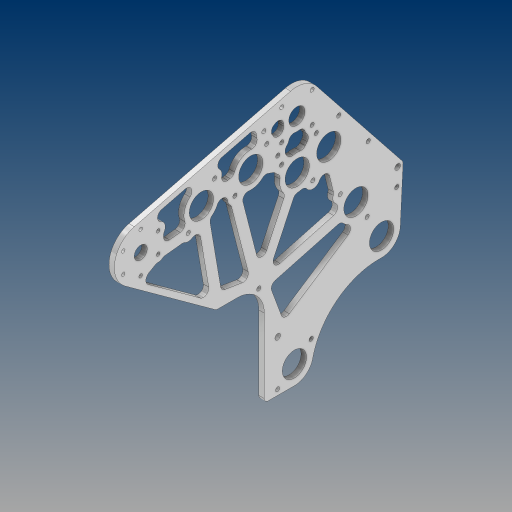
# Autodesk Inventor part: Intake Roller Plate
Saved by Autodesk Inventor 2024.3 (Build 283343000, 343)
## iProperties
Created: 2024-07-25
Part Number: Intake Roller Plate
Material: Aluminum 6061
Document SubType Name: Modeling
Designer: Kenji
Density: 2.7 g/cm^3
Appearance: Aluminum - Dark
Mass: 571.226 g
Surface Area: 904.797 cm^2
Volume: 211.565 cm^3
Author: Kenji
Autodesk Inventor part; units mm, degrees
ref_plane "YZ Plane" through (0, 0, 0) normal (1, 0, 0) x (0, 1, 0)
ref_plane "XZ Plane" through (0, 0, 0) normal (0, 1, 0) x (-1, 0, 0)
ref_plane "XY Plane" through (0, 0, 0) normal (0, 0, 1) x (1, 0, 0)
sketch "Sketch1" plane through (0, 0, 0) normal (1, 0, 0) x (0, 1, 0)
  line L0 (127, 0) -> (127, -31.75) construction
  line L1 (95.25, -63.5) -> (31.75, -63.5) construction
  line L2 (0, -31.75) -> (0, 0) construction
  arc A0 (95.25, -63.5) -> (127, -31.75) centre (95.25, -31.75) ccw construction
  arc A1 (0, -31.75) -> (31.75, -63.5) centre (31.75, -31.75) ccw construction
  line L3 (0, 0) -> (0, 19.05) construction
  line L4 (0, 19.05) -> (-12.7, 19.05) construction
  line L5 (82.55, 19.05) -> (82.55, 292.1) construction
  circle A2 centre (82.55, 292.1) radius 25.4 construction
  circle A3 centre (82.55, 292.1) radius 31.75 construction
  circle A4 centre (231.775, 292.1) radius 25.4 construction
  circle A5 centre (231.775, 292.1) radius 31.75 construction
  line L6 (-12.7, 19.05) -> (82.55, 19.05) construction
  line L7 (127, 0) -> (0, 0) construction
  line L8 (-12.7, 19.05) -> (-12.7, -285.75) construction
  circle A6 centre (38.1, -172.5837) radius 50.8 construction
  circle A7 centre (104.9083, -202.0677) radius 25.4 construction
  circle A8 centre (104.9083, -202.0677) radius 14.2875
  circle A9 centre (154.8209, -171.8196) radius 25.4 construction
  circle A10 centre (154.8209, -171.8196) radius 14.2875
  circle A11 centre (250.0002, -47.5843) radius 22.225 construction
  circle A12 centre (250.0002, -47.5843) radius 25.4 construction
  circle A13 centre (250.0002, -47.5843) radius 14.2875
  line L9 (82.55, 19.05) -> (127, 19.05) construction
  line L10 (127, 19.05) -> (127, 0) construction
  circle A14 centre (154.8209, -171.8196) radius 22.225 construction
  circle A15 centre (104.9083, -202.0677) radius 22.225 construction
  circle A16 centre (25.4, -99.06) radius 25.4 construction
  circle A17 centre (25.4, -99.06) radius 23.8125 construction
  line L11 (25.4, -73.66) -> (25.4, -63.5) construction
  circle A18 centre (219.8086, -102.3786) radius 25.4 construction
  circle A19 centre (219.8086, -102.3786) radius 22.225 construction
  circle A20 centre (219.8086, -102.3786) radius 14.2875
  line L12 (0, -99.06) -> (-12.7, -99.06) construction
  circle A21 centre (63.172, -79.375) radius 6.477 construction
  circle A22 centre (25.4, -99.06) radius 14.2875
  circle A23 centre (63.172, -79.375) radius 3.2512
  circle A24 centre (95.1707, -129.6948) radius 50.8 construction
  circle A25 centre (147.0613, -96.0158) radius 50.8 construction
  circle A26 centre (105.4747, -117.9903) radius 50.8 construction
  circle A27 centre (166.1747, -221.0415) radius 3.2512
  circle A28 centre (242.3971, 10.8357) radius 14.2875
  circle A29 centre (242.3971, 10.8357) radius 22.225 construction
  line L13 (219.8086, -102.3786) -> (154.8209, -171.8196) construction
  line L14 (154.8209, -171.8196) -> (104.9083, -202.0677) construction
  line L15 (82.55, 19.05) -> (31.75, 19.05) construction
  line L16 (31.75, 19.05) -> (31.75, 292.1) construction
  line L17 (31.75, 292.1) -> (82.55, 292.1) construction
  circle A30 centre (242.3971, 10.8357) radius 7.62 construction
  line L18 (-12.7, -285.75) -> (571.5, -285.75) construction
  line L19 (571.5, -285.75) -> (571.5, 292.1) construction
  line L20 (31.75, 292.1) -> (571.5, 292.1) construction
  line L21 (127, 19.05) -> (571.5, 19.05) construction
  circle A31 centre (230.3321, 82.55) radius 7.62
  circle A32 centre (230.3321, 82.55) radius 23.8125 construction
  circle A33 centre (254.1446, 82.55) radius 2.0828
  circle A34 centre (230.3321, 82.55) radius 27.94 construction
  circle A35 centre (230.3321, 82.55) radius 31.115 construction
  circle A36 centre (242.2384, 103.1722) radius 2.0828
  circle A37 centre (218.4259, 103.1722) radius 2.0828
  circle A38 centre (206.5196, 82.55) radius 2.0828
  circle A39 centre (218.4259, 61.9278) radius 2.0828
  circle A40 centre (242.2384, 61.9278) radius 2.0828
  line L22 (-12.7, -63.5) -> (368.3, -63.5) construction
  circle A41 centre (166.1747, -221.0415) radius 6.4262 construction
  line L23 (368.3, -63.5) -> (368.3, -285.75) construction
  circle A42 centre (63.172, -79.375) radius 6.35 construction
  circle A43 centre (242.3971, 10.8357) radius 25.4 construction
  line L24 (242.3971, 10.8357) -> (250.0002, -47.5843) construction
  line L25 (82.55, 19.05) -> (141.3002, 19.05) construction
  line L26 (141.3002, 19.05) -> (141.3002, 209.55) construction
  line L27 (141.3002, 209.55) -> (82.55, 209.55) construction
  line L28 (82.55, 209.55) -> (82.55, 19.05) construction
  circle A44 centre (133.35, 12.7) radius 6.35 construction
  circle A45 centre (177.4795, -39.017) radius 50.8 construction
  circle A46 centre (177.8, -23.221) radius 50.8 construction
  circle A47 centre (25.4, -99.06) radius 22.225 construction
  line L29 (3.175, -99.06) -> (3.175, -68.2752)
  circle A48 centre (133.35, 12.7) radius 3.2512 construction
  arc A49 (166.1747, -227.4677) -> (170.1786, -226.0679) centre (166.1747, -221.0415) ccw
  arc A50 (3.175, -99.06) -> (20.3984, -120.7149) centre (25.4, -99.06) ccw
  arc A51 (7.9502, -63.5) -> (3.175, -68.2752) centre (7.9502, -68.2752) ccw
  arc A52 (260.5134, 90.1152) -> (205.1617, 100.8419) centre (230.3321, 82.55) ccw
  line L30 (141.3002, 53.086) -> (157.9626, 53.086) construction
  line L31 (157.9626, 53.086) -> (157.9626, 86.106) construction
  line L32 (157.9626, 86.106) -> (141.3002, 86.106) construction
  line L33 (141.3002, 86.106) -> (141.3002, 53.086) construction
  line L34 (232.868, -28.832) -> (267.1324, -66.3365) construction
  circle A53 centre (232.868, -28.832) radius 2.4257
  circle A54 centre (267.1324, -66.3365) radius 2.4257
  line L35 (236.3587, 15.4834) -> (262.5254, -4.6567) construction
  line L36 (236.3587, 15.4834) -> (222.2689, 26.3281) construction
  circle A55 centre (262.5254, -4.6567) radius 2.4257
  circle A56 centre (222.2689, 26.3281) radius 2.4257
  circle A57 centre (262.5254, -4.6567) radius 6.35 construction
  circle A58 centre (222.2689, 26.3281) radius 6.35 construction
  circle A59 centre (232.868, -28.832) radius 6.35 construction
  circle A60 centre (267.1324, -66.3365) radius 6.35 construction
  line L37 (219.8086, -102.3786) -> (237.1646, -83.8332) construction
  line L38 (219.8086, -102.3786) -> (202.4526, -120.9239) construction
  circle A61 centre (237.1646, -83.8332) radius 2.4257
  circle A62 centre (202.4526, -120.9239) radius 2.4257
  circle A63 centre (172.1769, -153.2743) radius 2.4257
  circle A64 centre (133.0985, -184.9838) radius 2.4257
  arc A65 (82.6927, -201.4208) -> (103.7686, -224.2634) centre (104.9083, -202.0677) ccw
  circle A66 centre (9.525, -79.2321) radius 2.4257
  circle A67 centre (9.525, -79.2321) radius 6.35 construction
  arc A68 (82.6927, -201.4208) -> (20.3984, -120.7149) centre (2.2987, -199.0799) ccw
  line L39 (9.525, -79.2321) -> (41.275, -118.8879) construction
  circle A69 centre (41.275, -118.8879) radius 2.4257
  circle A70 centre (41.275, -118.8879) radius 5.6007 construction
  line L40 (7.9502, -63.5) -> (95.25, -63.5)
  arc A71 (95.25, -63.5) -> (127, -31.75) centre (95.25, -31.75) ccw
  line L41 (166.1747, -227.4677) -> (103.7686, -224.2634)
  line L42 (104.9083, -202.0677) -> (83.1859, -215.2319) construction
  line L43 (82.55, 133.35) -> (88.9, 133.35) construction
  line L44 (82.55, 184.15) -> (88.9, 184.15) construction
  line L45 (127, -31.75) -> (127, -8.2637)
  line L46 (127.9123, -5.4564) -> (205.1617, 100.8419)
  arc A72 (127.9123, -5.4564) -> (127, -8.2637) centre (131.7752, -8.2637) ccw
  line L47 (82.55, 44.45) -> (571.5, 44.45) construction
  circle A73 centre (133.0985, -184.9838) radius 6.35 construction
  circle A74 centre (141.7169, -99.98) radius 50.8 construction
  circle A75 centre (277.7476, -102.0288) radius 30 construction
  circle A76 centre (277.7476, -102.0288) radius 25.4 construction
  circle A77 centre (303.1476, -102.0288) radius 2.3876 construction
  circle A78 centre (295.7081, -84.0683) radius 2.3876
  circle A79 centre (277.7476, -76.6288) radius 2.3876 construction
  circle A80 centre (259.7871, -84.0683) radius 2.3876
  circle A81 centre (252.3476, -102.0288) radius 2.3876 construction
  circle A82 centre (259.7871, -119.9893) radius 2.3876
  circle A83 centre (277.7476, -127.4288) radius 2.3876 construction
  circle A84 centre (295.7081, -119.9893) radius 2.3876
  circle A85 centre (277.7476, -102.0288) radius 9.525
  circle A86 centre (219.8086, -102.3786) radius 19.05 construction
  circle A87 centre (227.4601, -139.7023) radius 19.05 construction
  circle A88 centre (227.4601, -139.7023) radius 14.2875
  line L48 (247.7482, -102.2099) -> (245.2082, -102.2252) construction
  line L49 (170.1786, -226.0679) -> (296.4391, -125.4942)
  line L50 (260.5134, 90.1152) -> (306.8474, -94.7347)
  arc A89 (296.4391, -125.4942) -> (306.8474, -94.7347) centre (277.7476, -102.0288) ccw
  circle A90 centre (219.8086, -102.3786) radius 30.48 construction
  circle A91 centre (277.7476, -102.0288) radius 30.48 construction
  circle A92 centre (248.6408, -79.4624) radius 3.81 construction
  line L51 (251.6519, -81.7968) -> (253.6592, -83.3531) construction
  line L52 (245.6582, -81.833) -> (243.6698, -83.4134) construction
  circle A93 centre (248.6408, -79.4624) radius 2.3812
  circle A94 centre (248.9154, -124.945) radius 3.81 construction
  circle A95 centre (248.9154, -124.945) radius 2.3876
  line L53 (251.898, -122.5744) -> (253.8865, -120.9939) construction
  line L54 (245.9043, -122.6105) -> (243.897, -121.0542) construction
  line L55 (248.6408, -75.6524) -> (248.6408, -72.9479) construction
  line L56 (219.8086, -102.3786) -> (219.8086, -88.0911) construction
  circle A96 centre (232.868, -28.832) radius 2.4257
  circle A97 centre (9.525, -79.2321) radius 2.4257
  circle A98 centre (146.08, -220.0775) radius 2.4257
  circle A99 centre (253.6387, -151.4689) radius 2.4257
  circle A100 centre (209.9304, -186.285) radius 2.4257
  circle A101 centre (281.6771, -62.9926) radius 2.4257
  line L57 (123.7263, -57.0623) -> (232.868, -28.832) construction
  line L58 (232.868, -28.832) -> (281.6771, -62.9926) construction
  line L59 (281.6771, -62.9926) -> (253.6387, -151.4689) construction
  line L60 (253.6387, -151.4689) -> (209.9304, -186.285) construction
  line L61 (209.9304, -186.285) -> (146.08, -220.0775) construction
  line L62 (146.08, -220.0775) -> (9.525, -79.2321) construction
  line L63 (123.7263, -57.0623) -> (9.525, -79.2321) construction
  circle A102 centre (146.08, -220.0775) radius 6.35 construction
  circle A103 centre (123.7263, -57.0623) radius 2.4257
  line L64 (277.7476, -102.0288) -> (219.8086, -102.3786) construction
  line L65 (250.0002, -47.5843) -> (219.8086, -102.3786) construction
  point P0 (-12.7, -172.5837)
  point P1 (180.2209, -171.8196)
  point P2 (104.775, 19.05)
  point P3 (172.6009, -221.0415)
  point P4 (127, -63.5)
  point P5 (3.175, -63.5)
  point P6 (104.9083, -227.4677)
  point P7 (95.25, -63.5)
  point P8 (127, -6.7118)
  point P9 (222.7121, 82.55)
  point P10 (220.1721, 10.8357)
  point P11 (25.4, -99.06)
  dimension "d58" = 101.6
  dimension "d267" = 15.24
  dimension "d283" = 15.24
  dimension "d284" = 47.625
  dimension "d523" = 50.8
  dimension "d2" = 31.75
  dimension "d3" = 19.05
  dimension "d4" = 12.7
  dimension "d7" = 273.05
  dimension "d8" = 50.8
  dimension "d9" = 6.35
  dimension "d10" = 50.8
  dimension "d11" = 6.35
  dimension "d12" = 149.225
  dimension "d14" = 127
  dimension "d16" = 304.8
  dimension "d175" = 31.75
  dimension "d180" = 50.8
  dimension "d181" = 1.5875
  dimension "d187" = 31.75
  dimension "d189" = 12.7
  dimension "d191" = 12.954
  dimension "d192" = 28.575
  dimension "d201" = 6.5024
  dimension "d207" = 101.6
  dimension "d208" = 101.6
  dimension "d210" = 130.175
  dimension "d214" = 15.875
  dimension "d218" = 6.5024
  dimension "d220" = 143.1895
  dimension "d236" = 50.8
  dimension "d237" = 44.45
  dimension "d271" = 584.2
  dimension "d285" = 4.1656
  dimension "d290" = 55.88
  dimension "d292" = 3.175
  dimension "d321" = 360
  dimension "d323" = 381
  dimension "d328" = 3.175
  dimension "d336" = 12.7
  dimension "d375" = 10.16
  dimension "d388" = 50.8
  dimension "d389" = 3.175
  dimension "d395" = 44.45
  dimension "d399" = 58.7502
  dimension "d400" = 190.5
  dimension "d404" = 12.7
  dimension "d405" = 101.6
  dimension "d406" = 101.6
  dimension "d409" = 3.175
  dimension "d410" = 6.5024
  dimension "d411" = 4.7752
  dimension "d427" = 16.6624
  dimension "d428" = 33.02
  dimension "d429" = 34.036
  dimension "d433" = 4.8514
  dimension "d434" = 4.8514
  dimension "d435" = 4.8514
  dimension "d436" = 4.8514
  dimension "d441" = 45
  dimension "d443" = 4.8514
  dimension "d444" = 4.8514
  dimension "d445" = 4.8514
  dimension "d446" = 4.8514
  dimension "d453" = 4.8514
  dimension "d459" = 4.8514
  dimension "d460" = 3.175
  dimension "d470" = 273.05
  dimension "d471" = 62.5615
  constraints: 133 end point, 97 centre point, 60 point on circle, 38 tangent, 36 point on line, 29 coincident, 16 equal radius, 16 perpendicular, 14 horizontal alignment, 12 concentric, 6 collinear, 6 horizontal, 6 parallel, 6 vertical, 5 midpoint, 4 equal length, 3 vertical alignment, 53 other
  measures "d2" radius of A0
  measures "d3" distance of L2.end L3.end
  measures "d4" distance of L3.end L4.end
  measures "d7" distance of L5.start L5.end
  measures "d8" diameter of A2
  measures "d9" radial gap between concentric circles of A2 A3
  measures "d10" diameter of A4
  measures "d11" radial gap between concentric circles of A4 A5
  measures "d12" distance of L17.end A4.centre
  measures "d14" distance of L0.start L2.end
  measures "d16" distance of L4.end L8.end
  measures "d175" radius of A1
  measures "d180" diameter of A16
  measures "d181" radial gap between concentric circles of A16 A17
  measures "d187" distance of L0.start L0.end
  measures "d189" distance of L12.start L12.end
  measures "d191" diameter of A21
  measures "d192" diameter of A22
  measures "d201" diameter of A23
  measures "d207" diameter of A24
  measures "d208" diameter of A25
  measures "d210" distance of A21.centre A14.centre
  measures "d214" distance from line of L1 A21.centre
  measures "d218" diameter of A27
  measures "d220" distance of A0.centre A19.centre
  measures "d236" distance of L5.start L15.end
  measures "d237" distance of L4.end L15.end
  measures "d271" distance of L8.end L18.end
  measures "d285" diameter of A33
  measures "d290" diameter of A34
  measures "d292" radial gap between concentric circles of A34 A35
  measures "d323" distance of L22.start L22.end
  measures "d328" radial gap between concentric circles of A27 A41
  measures "d336" diameter of A42
  measures "d375" distance of L11.start L11.end
  measures "d388" diameter of A9
  measures "d389" radial gap between concentric circles of A15 A7
  measures "d395" diameter of A15
  measures "d399" distance of L27.end L26.end
  measures "d400" distance of L26.end L25.end
  measures "d404" diameter of A44
  measures "d405" diameter of A45
  measures "d406" diameter of A46
  measures "d409" radial gap between concentric circles of A16 A47
  measures "d410" diameter of A48
  measures "d411" radius of A51
  measures "d427" distance of L32.end L31.end
  measures "d428" distance between parallel lines of L30 L32
  measures "d429" distance from line of L25.end L30
  measures "d433" diameter of A53
  measures "d434" diameter of A54
  measures "d435" diameter of A55
  measures "d436" diameter of A56
  measures "d441" angle of L24 L35
  measures "d443" diameter of A61
  measures "d444" diameter of A62
  measures "d445" diameter of A63
  measures "d446" diameter of A64
  measures "d453" diameter of A66
  measures "d459" diameter of A69
  measures "d460" radial gap between concentric circles of A69 A70
  measures "d470" distance of L19.end L21.end
  measures "d471" distance of A19.centre A11.centre
extrude "Extrusion14" add sketch "Sketch1" along normal blind 6.35 contours L29 A51 L40 A71 L45 A72 L46 A52 L50 A89 L49 A49 L41 A65 A68 A50 | A93 | A95 | A98 | A99 | A100 | A101 | A103
extrude "Extrusion16" cut sketch "Sketch1" along normal blind 6.35 contours A93 | A95
extrude "Extrusion17" cut sketch "Sketch1" along normal blind 25.4 contours A98 | A99 | A100 | A101 | A103
sketch "Sketch3" plane through (6.35, 0, 0) normal (1, 0, 0) x (0, 0, -1)
  circle A0 centre (151.4689, 253.6387) radius 2.4257 construction
  circle A1 centre (186.285, 209.9304) radius 2.4257 construction
  circle A2 centre (62.9926, 281.6771) radius 2.4257 construction
  circle A3 centre (220.0775, 146.08) radius 2.4257 construction
  circle A4 centre (57.0623, 123.7263) radius 2.4257 construction
  circle A5 centre (124.945, 248.9154) radius 2.3876 construction
  circle A6 centre (79.4624, 248.6408) radius 2.3812 construction
  line L0 (224.2634, 103.7686) -> (227.4677, 166.1747) projected
  arc A7 (227.4677, 166.1747) -> (226.0679, 170.1786) centre (221.0415, 166.1747) ccw projected
  line L1 (226.0679, 170.1786) -> (125.4942, 296.4391) projected
  arc A8 (125.4942, 296.4391) -> (94.7347, 306.8474) centre (102.0288, 277.7476) ccw projected
  line L2 (94.7347, 306.8474) -> (-90.1152, 260.5134) projected
  arc A9 (-90.1152, 260.5134) -> (-100.8419, 205.1617) centre (-82.55, 230.3321) ccw projected
  line L3 (-100.8419, 205.1617) -> (5.4564, 127.9123) projected
  arc A10 (5.4564, 127.9123) -> (8.2637, 127) centre (8.2637, 131.7752) ccw projected
  line L4 (8.2637, 127) -> (31.75, 127) projected
  arc A11 (63.5, 95.25) -> (31.75, 127) centre (31.75, 95.25) ccw projected
  line L5 (63.5, 95.25) -> (63.5, 7.9502) projected
  arc A12 (63.5, 7.9502) -> (68.2752, 3.175) centre (68.2752, 7.9502) ccw projected
  line L6 (68.2752, 3.175) -> (99.06, 3.175) projected
  arc A13 (99.06, 3.175) -> (120.7149, 20.3984) centre (99.06, 25.4) ccw projected
  arc A14 (201.4208, 82.6927) -> (120.7149, 20.3984) centre (199.0799, 2.2987) ccw projected
  arc A15 (201.4208, 82.6927) -> (224.2634, 103.7686) centre (202.0677, 104.9083) ccw projected
  circle A16 centre (119.9893, 259.7871) radius 2.3876 construction
  circle A17 centre (79.2321, 9.525) radius 2.4257 construction
  circle A18 centre (120.9239, 202.4526) radius 2.4257 construction
  circle A19 centre (-26.3281, 222.2689) radius 2.4257 construction
  circle A20 centre (28.832, 232.868) radius 2.4257 construction
  circle A21 centre (-61.9278, 242.2384) radius 2.0828 construction
  circle A22 centre (-61.9278, 218.4259) radius 2.0828 construction
  circle A23 centre (-82.55, 254.1446) radius 2.0828 construction
  circle A24 centre (-10.8357, 242.3971) radius 14.2875 construction
  circle A25 centre (79.375, 63.172) radius 3.2512 construction
  circle A26 centre (102.3786, 219.8086) radius 14.2875 construction
  circle A27 centre (171.8196, 154.8209) radius 14.2875 construction
  circle A28 centre (66.3365, 267.1324) radius 2.4257 construction
  circle A29 centre (83.8332, 237.1646) radius 2.4257 construction
  circle A30 centre (184.9838, 133.0985) radius 2.4257 construction
  circle A31 centre (118.8879, 41.275) radius 2.4257 construction
  circle A32 centre (139.7023, 227.4601) radius 14.2875 construction
  circle A33 centre (102.0288, 277.7476) radius 9.525 construction
  circle A34 centre (119.9893, 295.7081) radius 2.3876 construction
  circle A35 centre (84.0683, 259.7871) radius 2.3876 construction
  circle A36 centre (84.0683, 295.7081) radius 2.3876 construction
  circle A37 centre (153.2743, 172.1769) radius 2.4257 construction
  circle A38 centre (4.6567, 262.5254) radius 2.4257 construction
  circle A39 centre (-82.55, 206.5196) radius 2.0828 construction
  circle A40 centre (-103.1722, 218.4259) radius 2.0828 construction
  circle A41 centre (-103.1722, 242.2384) radius 2.0828 construction
  circle A42 centre (-82.55, 230.3321) radius 7.62 construction
  circle A43 centre (221.0415, 166.1747) radius 3.2512 construction
  circle A44 centre (99.06, 25.4) radius 14.2875 construction
  circle A45 centre (47.5843, 250.0002) radius 14.2875 construction
  circle A46 centre (202.0677, 104.9083) radius 14.2875 construction
  line L7 (120.5274, 292.4828) -> (221.1011, 166.2222) construction
  arc A47 (221.1109, 166.2061) -> (221.1011, 166.2222) centre (221.0415, 166.1747) ccw construction
  line L8 (221.1109, 166.2061) -> (217.9218, 104.0943) construction
  arc A48 (201.6056, 89.04) -> (217.9218, 104.0943) centre (202.0677, 104.9083) ccw construction
  arc A49 (201.6056, 89.04) -> (114.5278, 21.8275) centre (199.0799, 2.2987) ccw construction
  arc A50 (99.06, 9.525) -> (114.5278, 21.8275) centre (99.06, 25.4) ccw construction
  line L9 (99.06, 9.525) -> (69.85, 9.525) construction
  line L10 (69.85, 9.525) -> (69.85, 95.25) construction
  arc A51 (69.85, 95.25) -> (31.75, 133.35) centre (31.75, 95.25) ccw construction
  line L11 (31.75, 133.35) -> (8.7754, 133.35) construction
  line L12 (8.7754, 133.35) -> (-97.1089, 210.2985) construction
  arc A52 (-88.5712, 254.354) -> (-97.1089, 210.2985) centre (-82.55, 230.3321) ccw construction
  line L13 (-88.5712, 254.354) -> (96.2786, 300.6879) construction
  arc A53 (120.5274, 292.4828) -> (96.2786, 300.6879) centre (102.0288, 277.7476) ccw construction
  circle A54 centre (4.6567, 262.5254) radius 8.7757 construction
  circle A55 centre (-10.8357, 242.3971) radius 20.6375 construction
  circle A56 centre (-26.3281, 222.2689) radius 8.7757 construction
  circle A57 centre (-61.9278, 242.2384) radius 8.4328 construction
  circle A58 centre (-82.55, 254.1446) radius 8.4328 construction
  circle A59 centre (-61.9278, 218.4259) radius 8.4328 construction
  circle A60 centre (-82.55, 230.3321) radius 13.97 construction
  circle A61 centre (-82.55, 206.5196) radius 8.4328 construction
  circle A62 centre (-103.1722, 218.4259) radius 8.4328 construction
  circle A63 centre (-103.1722, 242.2384) radius 8.4328 construction
  circle A64 centre (47.5843, 250.0002) radius 20.6375 construction
  circle A65 centre (28.832, 232.868) radius 8.7757 construction
  circle A66 centre (62.9926, 281.6771) radius 8.7757 construction
  circle A67 centre (66.3365, 267.1324) radius 8.7757 construction
  circle A68 centre (102.0288, 277.7476) radius 15.875 construction
  circle A69 centre (84.0683, 259.7871) radius 8.7376 construction
  circle A70 centre (79.4624, 248.6408) radius 8.7312 construction
  circle A71 centre (83.8332, 237.1646) radius 8.7757 construction
  circle A72 centre (102.3786, 219.8086) radius 20.6375 construction
  circle A73 centre (120.9239, 202.4526) radius 8.7757 construction
  circle A74 centre (139.7023, 227.4601) radius 20.6375 construction
  circle A75 centre (124.945, 248.9154) radius 8.7376 construction
  circle A76 centre (119.9893, 259.7871) radius 8.7376 construction
  circle A77 centre (84.0683, 295.7081) radius 8.7376 construction
  circle A78 centre (119.9893, 295.7081) radius 8.7376 construction
  circle A79 centre (153.2743, 172.1769) radius 8.7757 construction
  circle A80 centre (171.8196, 154.8209) radius 20.6375 construction
  circle A81 centre (184.9838, 133.0985) radius 8.7757 construction
  circle A82 centre (57.0623, 123.7263) radius 8.7757 construction
  circle A83 centre (79.375, 63.172) radius 9.6012 construction
  line L14 (90.2467, 265.9655) -> (90.8035, 266.5223) construction
  line L15 (113.8109, 265.9655) -> (113.2541, 266.5223) construction
  line L16 (119.5913, 242.0101) -> (115.0235, 236.1184) construction
  line L17 (114.178, 245.3915) -> (111.9505, 242.5184)
  arc A84 (99.5909, 262.0609) -> (104.4667, 262.0609) centre (102.0288, 277.7476) ccw
  arc A85 (105.8607, 240.1502) -> (97.5577, 239.8752) centre (102.3786, 219.8086) ccw
  arc A86 (116.6652, 251.7065) -> (116.2491, 248.0628) centre (124.945, 248.9154) ccw construction
  arc A87 (111.5645, 257.4701) -> (113.7175, 253.7035) centre (119.9893, 259.7871) ccw
  arc A88 (90.1332, 253.4973) -> (92.4931, 257.4701) centre (84.0683, 259.7871) ccw
  arc A89 (88.182, 248.1918) -> (88.192, 248.806) centre (79.4624, 248.6408) ccw
  arc A90 (90.9354, 242.3195) -> (90.0356, 243.3729) centre (83.8332, 237.1646) ccw
  arc A91 (90.1332, 253.4973) -> (88.192, 248.806) centre (94.5409, 248.9262) ccw
  arc A92 (88.182, 248.1918) -> (90.0356, 243.3729) centre (94.5236, 247.8652) ccw
  arc A93 (90.9354, 242.3195) -> (97.5577, 239.8752) centre (96.0744, 246.0495) ccw
  arc A94 (105.8607, 240.1502) -> (111.9505, 242.5184) centre (106.9321, 246.4092) ccw
  arc A95 (114.178, 245.3915) -> (113.7175, 253.7035) centre (109.1596, 249.2822) ccw
  circle A96 centre (105.4418, 255.7862) radius 6.35 construction
  arc A97 (111.5645, 257.4701) -> (104.4667, 262.0609) centre (105.4418, 255.7862) ccw
  circle A98 centre (98.6158, 255.7862) radius 6.35 construction
  arc A99 (99.5909, 262.0609) -> (92.4931, 257.4701) centre (98.6158, 255.7862) ccw
  line L18 (144.6227, 207.4178) -> (151.182, 180.6995) construction
  line L19 (93.5751, 201.143) -> (60.8058, 131.6635) construction
  line L20 (87.3804, 68.4726) -> (177.6667, 128.2536) construction
  line L21 (76.0554, 72.1811) -> (60.0965, 115.4918) construction
  line L22 (97.964, 195.5626) -> (74.5331, 145.8831)
  line L23 (140.6011, 197.1653) -> (145.1487, 178.6417)
  line L24 (126.1934, 209.4701) -> (127.3102, 210.9574) construction
  arc A100 (103.3946, 199.1961) -> (107.1994, 199.7421) centre (102.3786, 219.8086) ccw
  arc A101 (113.8218, 197.2978) -> (128.7624, 198.5066) centre (120.9239, 202.4526) ccw
  arc A102 (113.8218, 197.2978) -> (107.1994, 199.7421) centre (108.6827, 193.5678) ccw
  arc A103 (103.3946, 199.1961) -> (97.964, 195.5626) centre (103.7073, 192.8538) ccw
  circle A104 centre (134.4342, 195.6513) radius 6.35 construction
  arc A105 (140.6011, 197.1653) -> (128.7624, 198.5066) centre (134.4342, 195.6513) ccw
  line L25 (151.9004, 149.4236) -> (65.5325, 126.0214) construction
  line L26 (150.4966, 142.4643) -> (76.4793, 122.4086)
  line L27 (93.1071, 79.8802) -> (162.4617, 125.8018)
  line L28 (83.643, 82.9793) -> (72.1817, 114.0841)
  arc A106 (76.4793, 122.4086) -> (72.1817, 114.0841) centre (78.1401, 116.2796) ccw
  arc A107 (83.643, 82.9793) -> (93.1071, 79.8802) centre (89.6014, 85.1748) ccw
  arc A108 (156.7838, 140.6848) -> (161.9828, 136.6786) centre (171.8196, 154.8209) ccw
  arc A109 (162.4617, 125.8018) -> (161.9828, 136.6786) centre (158.9561, 131.0964) ccw
  arc A110 (156.7838, 140.6848) -> (150.4966, 142.4643) centre (152.1573, 136.3353) ccw
  line L29 (70.2975, 286.5403) -> (76.7951, 290.866) construction
  line L30 (74.4441, 263.7739) -> (75.9959, 263.1311) construction
  line L31 (74.6662, 281.8202) -> (76.2852, 282.8981)
  line L32 (90.2467, 289.5297) -> (90.8035, 288.9729) construction
  arc A111 (86.1541, 277.651) -> (86.3421, 275.3097) centre (102.0288, 277.7476) ccw
  arc A112 (74.0356, 271.344) -> (73.2109, 272.5873) centre (66.3365, 267.1324) ccw
  arc A113 (69.1656, 275.4396) -> (71.5537, 279.7481) centre (62.9926, 281.6771) ccw construction
  arc A114 (74.6662, 281.8202) -> (73.2109, 272.5873) centre (78.1851, 276.5344) ccw
  circle A115 centre (79.8042, 277.6123) radius 6.35 construction
  circle A116 centre (80.0674, 274.3346) radius 6.35 construction
  arc A117 (86.1541, 277.651) -> (76.2852, 282.8981) centre (79.8042, 277.6123) ccw
  arc A118 (74.0356, 271.344) -> (86.3421, 275.3097) centre (79.8099, 274.5028) ccw
  line L33 (9.6292, 245.0605) -> (27.1194, 247.3368) construction
  line L34 (31.0296, 224.3719) -> (54.8647, 132.2224) construction
  line L35 (75.5608, 240.0938) -> (67.0382, 243.1117) construction
  line L36 (73.9692, 233.9211) -> (67.9115, 236.0661)
  line L37 (38.3043, 221.605) -> (54.4131, 159.326)
  line L38 (86.4774, 200.9801) -> (66.3041, 158.2074)
  arc A119 (76.8805, 231.8099) -> (79.1597, 229.7369) centre (83.8332, 237.1646) ccw
  arc A120 (82.037, 223.2908) -> (85.827, 207.4818) centre (102.3786, 219.8086) ccw
  arc A121 (45.189, 229.5022) -> (61.5078, 234.7673) centre (47.5843, 250.0002) ccw
  arc A122 (36.4965, 228.5939) -> (37.5607, 231.9604) centre (28.832, 232.868) ccw
  arc A123 (67.9115, 236.0661) -> (61.5078, 234.7673) centre (65.792, 230.0803) ccw
  arc A124 (76.8805, 231.8099) -> (73.9692, 233.9211) centre (71.8496, 227.9353) ccw
  arc A125 (82.037, 223.2908) -> (79.1597, 229.7369) centre (75.778, 224.3623) ccw
  arc A126 (86.4774, 200.9801) -> (85.827, 207.4818) centre (80.7342, 203.6889) ccw
  arc A127 (45.189, 229.5022) -> (38.3043, 221.605) centre (44.452, 223.1951) ccw
  arc A128 (54.4131, 159.326) -> (66.3041, 158.2074) centre (60.5608, 160.9161) ccw
  line L39 (-35.0531, 221.327) -> (-53.5437, 219.331) construction
  line L40 (-69.2308, 214.2095) -> (-75.247, 210.736) construction
  circle A129 centre (8.2637, 131.7752) radius 4.7752 construction
  line L41 (-7.3245, 222.0605) -> (7.4512, 136.4808) construction
  line L42 (-0.5269, 220.0122) -> (11.9246, 147.8939)
  line L43 (12.9752, 130.9981) -> (48.4036, 125.1545) construction
  line L44 (17.1486, 142.709) -> (37.2374, 139.3955)
  line L45 (24.7417, 223.324) -> (44.4185, 147.251)
  arc A130 (20.1011, 231.9826) -> (22.8921, 226.4081) centre (28.832, 232.868) ccw
  arc A131 (1.8326, 226.1054) -> (7.9908, 233.9431) centre (-10.8357, 242.3971) ccw
  arc A132 (37.2374, 139.3955) -> (44.4185, 147.251) centre (38.2708, 145.6608) ccw
  arc A133 (11.9246, 147.8939) -> (17.1486, 142.709) centre (18.1821, 148.9743) ccw
  arc A134 (1.8326, 226.1054) -> (-0.5269, 220.0122) centre (5.7305, 221.0926) ccw
  arc A135 (24.7417, 223.324) -> (22.8921, 226.4081) centre (18.594, 221.7338) ccw
  circle A136 centre (13.7835, 231.3419) radius 6.35 construction
  arc A137 (20.1011, 231.9826) -> (7.9908, 233.9431) centre (13.7835, 231.3419) ccw
  line L46 (2.523, 271.0377) -> (1.0727, 276.8239) construction
  line L47 (60.8589, 290.1895) -> (60.4768, 291.7139) construction
  line L48 (8.8186, 272.0384) -> (8.776, 272.2083)
  line L49 (20.218, 252.8422) -> (23.1514, 253.2239)
  line L50 (13.3916, 279.9117) -> (46.3266, 288.1671)
  arc A138 (13.2096, 260.5607) -> (10.645, 268.9404) centre (4.6567, 262.5254) ccw
  arc A139 (48.3753, 270.6226) -> (28.2736, 257.2807) centre (47.5843, 250.0002) ccw
  arc A140 (54.219, 281.8689) -> (54.6531, 278.9449) centre (62.9926, 281.6771) ccw
  arc A141 (23.1514, 253.2239) -> (28.2736, 257.2807) centre (22.3319, 259.5208) ccw
  arc A142 (8.8186, 272.0384) -> (10.645, 268.9404) centre (14.9781, 273.5823) ccw
  arc A143 (13.3916, 279.9117) -> (8.776, 272.2083) centre (14.9355, 273.7522) ccw
  circle A144 centre (48.6187, 276.9679) radius 6.35 construction
  circle A145 centre (47.8705, 282.0076) radius 6.35 construction
  arc A146 (48.3753, 270.6226) -> (54.6531, 278.9449) centre (48.6187, 276.9679) ccw
  arc A147 (54.219, 281.8689) -> (46.3266, 288.1671) centre (47.8705, 282.0076) ccw
  circle A148 centre (19.3984, 259.1391) radius 6.35 construction
  arc A149 (13.2096, 260.5607) -> (20.218, 252.8422) centre (19.3984, 259.1391) ccw
  line L51 (-35.785, 227.6349) -> (-48.5462, 226.2573)
  line L52 (-61.9278, 233.8056) -> (-61.9278, 226.8587) construction
  line L53 (-69.2308, 246.4548) -> (-75.247, 249.9282) construction
  line L54 (-55.5778, 234.6726) -> (-55.5778, 232.5706)
  line L55 (-57.8266, 262.0604) -> (-29.9386, 269.0507)
  arc A150 (-54.6831, 237.9225) -> (-58.7076, 250.0321) centre (-61.9278, 242.2384) ccw
  arc A151 (-27.9674, 230.8901) -> (-33.0319, 227.9321) centre (-26.3281, 222.2689) ccw construction
  arc A152 (-24.2631, 258.0691) -> (-30.4358, 235.9362) centre (-10.8357, 242.3971) ccw
  arc A153 (-35.785, 227.6349) -> (-30.4358, 235.9362) centre (-36.4666, 233.9482) ccw
  arc A154 (-55.5778, 232.5706) -> (-48.5462, 226.2573) centre (-49.2278, 232.5706) ccw
  arc A155 (-54.6831, 237.9225) -> (-55.5778, 234.6726) centre (-49.2278, 234.6726) ccw
  circle A156 centre (-56.2827, 255.9009) radius 6.35 construction
  circle A157 centre (-28.3947, 262.8912) radius 6.35 construction
  arc A158 (-24.2631, 258.0691) -> (-29.9386, 269.0507) centre (-28.3947, 262.8912) ccw
  arc A159 (-57.8266, 262.0604) -> (-58.7076, 250.0321) centre (-56.2827, 255.9009) ccw
  line L56 (-33.8148, 215.0738) -> (-53.7242, 212.9246)
  line L57 (-65.3049, 209.1437) -> (-72.8228, 204.8033)
  arc A160 (-62.0431, 209.9939) -> (-56.8593, 211.6863) centre (-61.9278, 218.4259) ccw
  arc A161 (-30.2763, 214.4315) -> (-21.5319, 214.9198) centre (-26.3281, 222.2689) ccw
  line L58 (-11.804, 210.6824) -> (-2.15, 154.7672)
  line L59 (-73.8457, 193.3926) -> (-12.1404, 148.55)
  arc A162 (-75.4551, 201.9617) -> (-75.19, 202.4035) centre (-82.55, 206.5196) ccw
  arc A163 (-12.1404, 148.55) -> (-2.15, 154.7672) centre (-8.4074, 153.6869) ccw
  arc A164 (-53.7242, 212.9246) -> (-56.8593, 211.6863) centre (-53.0426, 206.6113) ccw
  arc A165 (-30.2763, 214.4315) -> (-33.8148, 215.0738) centre (-33.1332, 208.7605) ccw
  arc A166 (-62.0431, 209.9939) -> (-65.3049, 209.1437) centre (-62.1299, 203.6445) ccw
  arc A167 (-72.8228, 204.8033) -> (-75.19, 202.4035) centre (-69.6478, 199.304) ccw
  arc A168 (-75.4551, 201.9617) -> (-73.8457, 193.3926) centre (-70.1126, 198.5295) ccw
  circle A169 centre (-18.0614, 209.6021) radius 6.35 construction
  arc A170 (-11.804, 210.6824) -> (-21.5319, 214.9198) centre (-18.0614, 209.6021) ccw
  line L60 (145.4601, 154.2575) -> (81.9371, 137.0454)
  arc A171 (144.982, 175.0493) -> (147.7771, 165.3363) centre (153.2743, 172.1769) ccw
  arc A172 (74.5331, 145.8831) -> (81.9371, 137.0454) centre (80.2764, 143.1743) ccw
  arc A173 (144.982, 175.0493) -> (145.1487, 178.6417) centre (138.9818, 177.1277) ccw
  circle A174 centre (143.7994, 160.3865) radius 6.35 construction
  arc A175 (145.4601, 154.2575) -> (147.7771, 165.3363) centre (143.7994, 160.3865) ccw
  point P0 (0, 0)
  point P1 (109.3917, 239.218)
  point P2 (99.7455, 199.3398)
  point P3 (145.6633, 176.5455)
  point P4 (68.6693, 133.4503)
  point P5 (154.5275, 143.5565)
  point P6 (175.6667, 134.5451)
  point P7 (76.0038, 233.2006)
  point P8 (63.9748, 237.46)
  point P9 (88.2589, 204.7573)
  point P10 (-1.2374, 224.1275)
  point P11 (24.2012, 225.4136)
  point P12 (9.3434, 269.9448)
  point P13 (7.2321, 278.3678)
  point P14 (27.2927, 253.7629)
  point P15 (-55.5778, 236.6895)
  point P16 (-31.6688, 215.3055)
  point P17 (-55.7295, 212.7081)
  point P18 (-63.5582, 210.1522)
  point P19 (-74.5696, 203.7948)
  point P20 (-80.6148, 198.3119)
  point P21 (54.6531, 278.9449)
  dimension "d656" = 12.7
  dimension "d596" = 6.35
  dimension "d597" = 6.35
  dimension "d598" = 6.35
  dimension "d599" = 6.35
  dimension "d600" = 6.35
  dimension "d601" = 6.35
  dimension "d602" = 6.35
  dimension "d603" = 6.35
  dimension "d604" = 6.35
  dimension "d605" = 6.35
  dimension "d606" = 6.35
  dimension "d607" = 6.35
  dimension "d608" = 6.35
  dimension "d609" = 6.35
  dimension "d610" = 6.35
  dimension "d611" = 6.35
  dimension "d612" = 6.35
  dimension "d613" = 6.35
  dimension "d614" = 6.35
  dimension "d615" = 6.35
  dimension "d616" = 6.35
  dimension "d617" = 6.35
  dimension "d618" = 6.35
  dimension "d619" = 6.35
  dimension "d620" = 6.35
  dimension "d621" = 6.35
  dimension "d622" = 6.35
  dimension "d623" = 6.35
  dimension "d624" = 6.35
  dimension "d625" = 6.35
  dimension "d626" = 6.35
  dimension "d629" = 6.35
  dimension "d630" = 6.35
  dimension "d631" = 6.35
  dimension "d632" = 6.35
  dimension "d633" = 6.35
  dimension "d635" = 12.7
  dimension "d636" = 12.7
  dimension "d637" = 6.35
  dimension "d638" = 6.35
  dimension "d642" = 6.35
  dimension "d643" = 12.7
  dimension "d645" = 6.35
  dimension "d646" = 6.35
  dimension "d648" = 6.35
  dimension "d649" = 6.35
  dimension "d650" = 6.35
  dimension "d654" = 6.35
  dimension "d655" = 12.7
  dimension "d657" = 6.35
  dimension "d658" = 6.35
  dimension "d659" = 6.35
  dimension "d660" = 6.35
  dimension "d661" = 6.35
  dimension "d663" = 6.35
  dimension "d665" = 6.35
  dimension "d666" = 6.35
  dimension "d667" = 6.35
  dimension "d668" = 12.7
  dimension "d669" = 6.35
  dimension "d670" = 6.35
  dimension "d672" = 6.35
  dimension "d673" = 6.35
  dimension "d674" = 6.35
  constraints: 298 point on circle, 125 centre point, 111 tangent, 108 end point, 78 point on line, 44 concentric, 21 parallel, 15 equal radius, 2 collinear, 2 perpendicular, 1 coincident, 34 other
  measures "d596" distance between parallel lines of L1 L7
  measures "d597" radial gap between concentric circles of A38 A54
  measures "d598" radial gap between concentric circles of A24 A55
  measures "d599" radial gap between concentric circles of A19 A56
  measures "d600" radial gap between concentric circles of A21 A57
  measures "d602" radial gap between concentric circles of A22 A59
  measures "d603" radial gap between concentric circles of A42 A60
  measures "d604" radial gap between concentric circles of A39 A61
  measures "d605" radial gap between concentric circles of A40 A62
  measures "d606" radial gap between concentric circles of A41 A63
  measures "d607" radial gap between concentric circles of A45 A64
  measures "d608" radial gap between concentric circles of A20 A65
  measures "d609" radial gap between concentric circles of A2 A66
  measures "d610" radial gap between concentric circles of A28 A67
  measures "d612" radial gap between concentric circles of A35 A69
  measures "d613" radial gap between concentric circles of A6 A70
  measures "d614" radial gap between concentric circles of A29 A71
  measures "d615" radial gap between concentric circles of A26 A72
  measures "d616" radial gap between concentric circles of A18 A73
  measures "d617" radial gap between concentric circles of A32 A74
  measures "d618" radial gap between concentric circles of A5 A75
  measures "d619" radial gap between concentric circles of A16 A76
  measures "d620" radial gap between concentric circles of A36 A77
  measures "d621" radial gap between concentric circles of A34 A78
  measures "d622" radial gap between concentric circles of A37 A79
  measures "d623" radial gap between concentric circles of A27 A80
  measures "d625" radial gap between concentric circles of A4 A82
  measures "d626" radial gap between concentric circles of A25 A83
  measures "d629" distance between parallel lines of L16 L17
  measures "d630" radius of A91
  measures "d631" radius of A92
  measures "d632" radius of A93
  measures "d633" radius of A95
  measures "d635" diameter of A96
  measures "d636" diameter of A98
  measures "d637" distance between parallel lines of L19 L22
  measures "d638" distance between parallel lines of L18 L23
  measures "d642" radius of A102
  measures "d643" diameter of A104
  measures "d645" distance between parallel lines of L25 L26
  measures "d646" distance between parallel lines of L20 L27
  measures "d648" radius of A106
  measures "d649" radius of A109
  measures "d650" distance between parallel lines of L29 L31
  measures "d654" radius of A114
  measures "d655" diameter of A115
  measures "d657" distance between parallel lines of L35 L36
  measures "d658" distance between parallel lines of L34 L37
  measures "d659" distance between parallel lines of L19 L38
  measures "d660" radius of A123
  measures "d661" radius of A127
  measures "d663" distance between parallel lines of L41 L42
  measures "d665" distance between parallel lines of L34 L45
  measures "d666" radius of A132
  measures "d667" radius of A135
  measures "d668" diameter of A136
  measures "d669" distance between parallel lines of L46 L48
  measures "d670" distance between parallel lines of L33 L49
  measures "d672" radius of A141
  measures "d673" radius of A142
  measures "d674" radius of A143
extrude "Extrusion21" cut sketch "Sketch3" against normal blind 25.4 contours L17 A94 A85 A93 A90 A92 A89 A91 A88 A99 A84 A97 A87 A95 | A103 A100 A102 A101 A105 L23 A173 A171 A175 L60 A172 L22 | A110 A108 A109 L27 A107 L28 A106 L26 | L31 A117 A111 A118 A112 A114 | A124 A119 A125 A120 A126 L38 A128 L37 A127 A121 A123 L36 | A134 A131 A137 A130 A135 L45 A132 L44 A133 L42 | L48 A143 L50 A147 A140 A146 A139 A141 L49 A149 A138 A142 | L51 A154 L54 A155 A150 A159 L55 A158 A152 A153 | A165 A161 A170 L58 A163 L59 A168 A162 A167 L57 A166 A160 A164 L56
body "Solid13"
